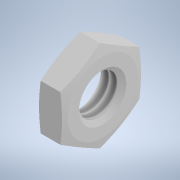
# Autodesk Inventor part: ISO 4035 M6(F)
Saved by Autodesk Inventor 2021 (Build 250183000, 183)
## iProperties
Created: 2026-04-25
Part Number: ISO 4035 M6(F)
Material: Generic
Catalog Web Link: www.3dfindit.com
Description: ISO 4035-Hexagon thin nuts (chamfered) - Product grades A and B
Vendor: FESTO
Document SubType Name: Modeling
Designer: psAdmin
Manufacturer: FESTO
Mass: 0.205666 g
Surface Area: 2.73059 cm^2
Volume: 0.205666 cm^3
Density: 1 g/cm^3
Appearance: PSOLRGB-176-176-176
Category: PARTsolutions
Company: FESTO
Title: ISO 4035 M6(F)
Author: Cadenas PARTsolutions
Comments: Hexagon thin nuts (chamfered) - Product grades A and B
PSOL_IDENT_0: {$CADENAS_DATA/23d-libs/festo/zyl_zubeh/iso_4035/din_iso_4035.prj},171 {VTYP=3D},{NB=ISO 4035 M6(F)}
PSOL_IDENT_1: ,{LINA=ISO 4035 M6(F)},{NN=ISO 4035},{DATE=13.09.2023 12:11:15},{GEOMDATE=13.09.2023 12:10:57},{VERS
PSOL_IDENT_2: ION=},{LINEID=320},{WBVAR=},{WBNUMERIC=}  {NB=ISO 4035 M6(F)},{LINA=ISO 4035 M6(F)},{KT=X},{IDNR=},{
PSOL_IDENT_3: NENN=M6},{D=6.000},{D1=4.917},{P=1.000},{D2=8.900},{E=11.050},{M=3.200},{S=10.000},{CNSAVOID=0},{DIS
PSOL_IDENT_4: T=0.407143}
NB: ISO 4035 M6(F)
NN: ISO 4035
NT: Hexagon thin nuts (chamfered) - Product grades A and B
NBSYN: ISO 4035 $NENN.(F)
LINA: ISO 4035 M6(F)
CATALOG: Festo
ROWDESC: M6
NENN: M6
D: 6
D1: 4.917
P: 1
D2: 8.9
E: 11.05
M: 3.2
S: 10
SUPPLIER: FESTO
ARTICLENO: ISO 4035 M6(F)
BOMINFO: ISO 4035 M6(F)
CREATOR: CADENAS GmbH
Autodesk Inventor part; units mm, degrees
sketch "Sketch_1" plane through (0, 0, 0) normal (0, 1, 0) x (-1, 0, 0)
  line L0 (-3.2, 0) -> (0, 0)
  line L1 (0, 0) -> (0, -6)
  line L2 (0, -6) -> (-3.2, -6)
  line L3 (-3.2, -6) -> (-3.2, 0)
  line L4 (-3.2, 0) -> (0, 0)
  constraints: 10 end point
revolve "Revolution1" add sketch "Sketch_1" angle 360 about axis through (3.2, 0, 0) along (1, 0, 0)
sketch "Sketch_3" plane through (0, 0, 0) normal (0, 0, 1) x (1, 0, 0)
  line L0 (3.2, 0) -> (0, 0)
  line L1 (-4.45, 10) -> (-4.45, 4.45)
  line L2 (-4.45, 4.45) -> (0, 4.45)
  line L3 (0, 4.45) -> (0.4153, 6)
  line L4 (0.4153, 6) -> (2.7847, 6)
  line L5 (2.7847, 6) -> (3.2, 4.45)
  line L6 (3.2, 4.45) -> (7.65, 4.45)
  line L7 (7.65, 4.45) -> (7.65, 10)
  line L8 (7.65, 10) -> (-4.45, 10)
  constraints: 18 end point
revolve "Revolution2" cut sketch "Sketch_3" angle 360 about axis through (3.2, 0, 0) along (1, 0, 0)
sketch "Skizze_3" plane through (0, 0, 0) normal (0, 0, 1) x (1, 0, 0)
  line L0 (3.2, 0) -> (0, 0)
  line L1 (0, 0) -> (0, 3)
  line L2 (0, 3) -> (0.5415, 2.4585)
  line L3 (0.5415, 2.4585) -> (2.6585, 2.4585)
  line L4 (2.6585, 2.4585) -> (3.2, 3)
  line L5 (3.2, 3) -> (3.2, 0)
  line L6 (3.2, 0) -> (0, 0)
  constraints: 14 end point
revolve "Revolution3" cut sketch "Skizze_3" angle 360 about axis through (3.2, 0, 0) along (1, 0, 0)
thread "Thread1" size "M6x1" class "6H" standard "ISO Metric profile" full length
sketch "Sketch_2" plane through (0, 0, 0) normal (1, 0, 0) x (0, 1, 0)
  line L0 (20, 20) -> (-20, 20)
  line L1 (-20, 20) -> (-20, -20)
  line L2 (-20, -20) -> (20, -20)
  line L3 (20, -20) -> (20, 20)
  line L4 (2.8868, 5) -> (-2.8868, 5)
  line L5 (-2.8868, 5) -> (-5.7735, 0)
  line L6 (-5.7735, 0) -> (-2.8868, -5)
  line L7 (-2.8868, -5) -> (2.8868, -5)
  line L8 (2.8868, -5) -> (5.7735, 0)
  line L9 (5.7735, 0) -> (2.8868, 5)
  constraints: 20 end point
extrude "Extrusion1" cut sketch "Sketch_2" along normal mid plane 8.4
ref_plane "2CYL_XY" through (1.6, 0, 0) normal (1, 0, 0) x (0, 0, -1)
ref_plane "2CYL_YZ" through (1.6, 0, 0) normal (0, 0, -1) x (0, 1, 0)
ref_plane "2CYL_ZX" through (1.6, 0, 0) normal (0, 1, 0) x (1, 0, 0)
ref_plane "IP1_XY" through (0, 0, 0) normal (1, 0, 0) x (0, 0, -1)
ref_plane "IP1_YZ" through (0, 0, 0) normal (0, 0, -1) x (0, 1, 0)
ref_plane "IP1_ZX" through (0, 0, 0) normal (0, 1, 0) x (1, 0, 0)
ref_plane "IP2_XY" through (3.2, 0, 0) normal (1, 0, 0) x (0, 0, -1)
ref_plane "IP2_YZ" through (3.2, 0, 0) normal (0, 0, -1) x (0, 1, 0)
ref_plane "IP2_ZX" through (3.2, 0, 0) normal (0, 1, 0) x (1, 0, 0)
body "Solid1"
